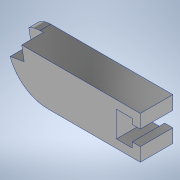
# Autodesk Inventor part: Finray_test_8_Kerbe_10deg_V4_links
Saved by Autodesk Inventor 2022 (Build 260153000, 153)
## iProperties
Created: 2022-02-28
Part Number: Finray_test_8_Kerbe_10deg_V4_links
Material: Generic
Document SubType Name: Modeling
Designer: richa
Density: 1 g/cm^3
Appearance: Aluminum - Flat
Author: richa
Autodesk Inventor part; units mm, degrees
ref_plane "YZ Plane" through (0, 0, 0) normal (1, 0, 0) x (0, 1, 0)
ref_plane "XZ Plane" through (0, 0, 0) normal (0, 1, 0) x (-1, 0, 0)
ref_plane "XY Plane" through (0, 0, 0) normal (0, 0, 1) x (1, 0, 0)
sketch "Sketch5" plane through (0, 0, 0) normal (0, 0, 1) x (1, 0, 0)
  line L0 (52.8, -15.6) -> (52.8, -10.6)
  line L1 (52.8, -10.6) -> (49.8, -10.6)
  line L2 (49.8, -10.6) -> (49.8, -12.55)
  line L3 (44, -12.55) -> (44, -3.05)
  line L4 (49.8, -3.05) -> (49.8, -5)
  line L5 (49.8, -5) -> (52.8, -5)
  line L6 (52.8, -5) -> (52.8, 0)
  line L7 (52.8, 0) -> (7.8, 0)
  line L8 (44, -3.05) -> (49.8, -3.05)
  line L9 (44, -12.55) -> (49.8, -12.55)
  line L10 (52.8, -15.6) -> (7.8, -15.6)
  arc A0 (7.8, 0) -> (7.8, -15.6) centre (7.8, -7.8) ccw
  point P0 (0, 0)
  dimension "d41" = 5.8
  dimension "d48" = 44
  dimension "d50" = 3
  dimension "d63" = 45
  dimension "d67" = 15.6
  dimension "d71" = 0
  dimension "d72" = 36.2
  dimension "d87" = 5.6
  dimension "d88" = 9.5
  constraints: 22 end point, 7 perpendicular, 4 collinear, 2 parallel, 2 point on circle, 2 tangent, 1 centre point, 1 horizontal, 1 vertical
  measures "d41" distance between parallel lines of L2 L3
  measures "d48" distance from line of L3 point (0, 0)
  measures "d50" distance of L4.end L5.end
  measures "d63" distance of L0.start L10.end
  measures "d67" diameter of A0
  measures "d71" distance from line of point (0, 0) L7
  measures "d72" distance from line of L3 A0.centre
  measures "d87" distance from line of L0.end L5
  measures "d88" distance of L3.start L3.end
extrude "Extrusion2" add sketch "Sketch5" along normal blind 12
sketch "Sketch11" plane through (0, 0, 12) normal (0, 0, 1) x (1, 0, 0)
  line L0 (52.8, 0) -> (7.8, 0) projected
  line L1 (9.0635, 0) -> (9.9318, -4.924)
  line L2 (9.9318, -4.924) -> (0.0837, -6.6605)
  arc A0 (7.8, 0) -> (7.8, -15.6) centre (7.8, -7.8) ccw projected
  point P0 (0, 0)
  dimension "d95" = 100
  dimension "d96" = 5
  dimension "d97" = 10
  constraints: 4 end point, 1 perpendicular, 1 point on circle, 1 point on line
  measures "d95" angle of L0 L1
  measures "d96" distance of L1.start L1.end
  measures "d97" distance of L1.end L2.end
extrude "Extrusion7" cut sketch "Sketch11" against normal blind 8 from surface at 0
sketch "Sketch14" plane through (0, 0, 12) normal (0, 0, 1) x (1, 0, 0)
  line L0 (2.6339, 4.7908) -> (6.9247, -19.5432)
  line L1 (6.9247, -19.5432) -> (-9.4392, -22.4286)
  line L2 (-9.4392, -22.4286) -> (-13.7299, 1.9055)
  line L3 (-13.7299, 1.9055) -> (2.6339, 4.7908)
  line L4 (9.0635, 0) -> (9.9318, -4.924) projected
  point P0 (0, 0)
  dimension "d107" = 5.5
  constraints: 8 end point, 2 parallel, 2 perpendicular
  measures "d107" distance between parallel lines of L0 L4
extrude "Extrusion10" cut sketch "Sketch14" against normal through all
fillet "Fillet2" radius 15 1 edges at (6.2001, -15.4342, 6)
equation "\"l1\" = 8"
body "Solid2"
